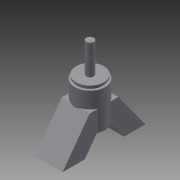
# Autodesk Inventor part: gear mount
Saved by Autodesk Inventor 2015 (Build 190159000, 159)
## iProperties
Created: 2015-03-26
Part Number: gear mount
Material: Generic
Document SubType Name: Modeling
Designer: WASHHSST
Density: 1 g/cm^3
Appearance: Default
Author: WASHHSST
Autodesk Inventor part; units mm, degrees
ref_plane "YZ Plane" through (0, 0, 0) normal (1, 0, 0) x (0, 1, 0)
ref_plane "XZ Plane" through (0, 0, 0) normal (0, 1, 0) x (-1, 0, 0)
ref_plane "XY Plane" through (0, 0, 0) normal (0, 0, 1) x (1, 0, 0)
sketch "Sketch3" plane through (0, 0, 0) normal (1, 0, 0) x (0, 1, 0)
  line L0 (0, -27.432) -> (0, -56.388)
  line L1 (0, -56.388) -> (50.8, -19.4796)
  line L2 (50.8, -19.4796) -> (50.8, 9.4764)
  line L3 (7.4884, -44.196) -> (-9.6833, -44.196) construction
  line L4 (0, -27.432) -> (50.8, 9.4764)
  line L5 (0, 56.388) -> (50.8, 19.4796)
  line L6 (50.8, 19.4796) -> (50.8, -10.7464)
  line L7 (0, 56.388) -> (0, 26.162)
  line L8 (0, 26.162) -> (50.8, -10.7464)
  point P0 (0, 0)
  dimension "d23" = 54
  dimension "d25" = 44.196
  dimension "d26" = 16.764
  dimension "d27" = 12.192
  dimension "d28" = 50.8
  dimension "d33" = 0
  dimension "d34" = 54
  dimension "d35" = 50.8
  dimension "d36" = 53.594
  dimension "d37" = 112.776
  constraints: 19 end point, 3 vertical, 1 collinear, 1 horizontal, 1 parallel
  measures "d23" angle of L0 L1
  measures "d25" vertical distance of L3.end point (0, 0)
  measures "d26" distance from line of L3 L0.start
  measures "d27" distance from line of L0.end L3
  measures "d28" distance between parallel lines of L0 L2
  measures "d33" horizontal distance of point (0, 0) L0.end
  measures "d34" angle of L7 L5
  measures "d35" distance between parallel lines of L7 L6
  measures "d36" distance of L0.start L7.end
  measures "d37" distance of L0.end L5.start
extrude "Extrusion1" add sketch "Sketch3" along normal blind 38.1
sketch "Sketch5" plane through (0, 50.8, 19.4796) normal (0, 1, 0) x (1, 0, 0)
  circle A0 centre (19.05, 19.4775) radius 20.701
  line L0 (0, 38.9593) -> (38.1, 38.9593) projected
  line L1 (38.1, 38.9593) -> (38.1, 0) projected
  line L2 (0, 0) -> (38.1, 0) projected
  line L3 (38.1, 0) -> (0, 0) projected
  line L4 (0, 0) -> (0, 38.9593) projected
  line L5 (0, 38.9593) -> (38.1, 38.9593) projected
  line L6 (38.1, 38.9593) -> (38.1, 0) projected
  point P0 (0, 19.4796)
  dimension "d40" = 41.402
  dimension "d42" = 19.05
  dimension "d43" = 38.9593
  dimension "d44" = 19.4818
  constraints: 1 centre point
  measures "d40" diameter of A0
  measures "d42" distance from line of A0.centre L1
  measures "d43" distance from line of L2 L0.start
  measures "d44" distance from line of L0 A0.centre
extrude "Extrusion2" add sketch "Sketch5" along normal blind 22.098 contours A0 L1 | L1 A0 L2 L4 L0 | L0 A0 | A0 L2 | L4 A0
extrude "Extrusion3" add sketch "Sketch5" against normal blind 28.448 contours A0 L1 | L1 A0 L2 L4 L0 | L0 A0 | A0 L2 | L4 A0
sketch "Sketch8" plane through (19.05, 72.898, 0.0022) normal (0, 1, 0) x (1, 0, 0)
  circle A0 centre (0, 0) radius 17.526
  circle A1 centre (0, 0) radius 20.701 projected
  point P0 (-19.05, 0.0022)
  dimension "d50" = 35.052
  constraints: 1 centre point, 1 concentric
  measures "d50" diameter of A0
extrude "Extrusion4" add sketch "Sketch8" along normal blind 2.54 contours A0
sketch "Sketch9" plane through (19.05, 75.438, 0.0022) normal (0, 1, 0) x (1, 0, 0)
  circle A0 centre (0, 0) radius 19.05
  circle A1 centre (0, 0) radius 17.526 projected
  point P0 (-19.05, 0.0022)
  dimension "d53" = 38.1
  constraints: 1 centre point, 1 concentric
  measures "d53" diameter of A0
extrude "Extrusion5" add sketch "Sketch9" along normal blind 2.286 contours A0 | A1
sketch "Sketch10" plane through (19.05, 77.724, 0.0022) normal (0, 1, 0) x (1, 0, 0)
  circle A0 centre (0, 0) radius 5.08
  circle A1 centre (0, 0) radius 19.05 projected
  point P0 (-19.05, 0.0022)
  dimension "d56" = 10.16
  constraints: 1 centre point, 2 other
  measures "d56" diameter of A0
extrude "Extrusion6" add sketch "Sketch10" along normal blind 40.64 contours A0
body "Solid1"
